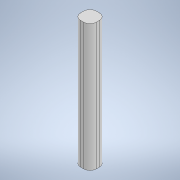
# Autodesk Inventor part: Noga
Saved by Autodesk Inventor 2021 (Build 250183000, 183)
## iProperties
Created: 2020-04-11
Part Number: Noga
Material: Ogólny
Document SubType Name: Modeling
Designer: dyrag
Density: 1 g/cm^3
Appearance: Domyślna
Author: dyrag
Autodesk Inventor part; units mm, degrees
ref_plane "YZ Plane" through (0, 0, 0) normal (1, 0, 0) x (0, 1, 0)
ref_plane "XZ Plane" through (0, 0, 0) normal (0, 1, 0) x (-1, 0, 0)
ref_plane "XY Plane" through (0, 0, 0) normal (0, 0, 1) x (1, 0, 0)
sketch "Szkic1" plane through (0, 0, 0) normal (0, 0, 1) x (1, 0, 0)
  line L0 (0, 0) -> (0, 40)
  line L1 (0, 40) -> (5, 40)
  line L2 (5, 40) -> (5, 0)
  line L3 (5, 0) -> (0, 0)
  dimension "d0" = 40
  dimension "d1" = 5
  constraints: 8 end point, 3 perpendicular, 1 vertical
  measures "d0" distance of L0.start L0.end
  measures "d1" distance of L0.end L1.end
extrude "Wyciągnięcie proste1" add sketch "Szkic1" along normal blind 5
fillet "Zaokrąglenie1" radius 2 4 edges at (5, 20, 5) (5, 20, 0) (0, 20, 0) (0, 20, 5)
